Autodesk Fusion 360 part; units mm, degrees
(part 4 of 5)
  spline S117 degree 5 poles (-17.8005, -20.6587) (-17.8021, -20.6614) (-17.8082, -20.6716) (-17.8187, -20.6895) (-17.8335, -20.715) (-17.8525, -20.7483) (-17.8741, -20.7867) (-17.8954, -20.8254) (-17.9164, -20.8642) (-17.9371, -20.9032) (-17.9576, -20.9425) (-17.9778, -20.9819) (-17.9978, -21.0215) (-18.0175, -21.0613) (-18.037, -21.1012) (-18.0562, -21.1414) (-18.0753, -21.1816) (-18.0941, -21.2221) (-18.1127, -21.2627) (-18.1311, -21.3034) (-18.1492, -21.3443) (-18.1672, -21.3853) (-18.1849, -21.4265) (-18.2025, -21.4679) (-18.2198, -21.5093) (-18.237, -21.5509) (-18.2539, -21.5926) (-18.2706, -21.6345) (-18.2872, -21.6765) (-18.3036, -21.7186) (-18.3198, -21.7608) (-18.3357, -21.8032) (-18.3516, -21.8457) (-18.3672, -21.8882) (-18.3826, -21.931) (-18.3979, -21.9738) (-18.413, -22.0167) (-18.4279, -22.0598) (-18.4426, -22.103) (-18.4571, -22.1462) (-18.4715, -22.1896) (-18.4857, -22.2331) (-18.4998, -22.2767) (-18.5136, -22.3204) (-18.5273, -22.3642) (-18.5409, -22.4081) (-18.5542, -22.4521) (-18.5674, -22.4962) (-18.5805, -22.5404) (-18.5933, -22.5847) (-18.606, -22.6291) (-18.6186, -22.6736) (-18.6309, -22.7182) (-18.6432, -22.7628) (-18.6552, -22.8076) (-18.6671, -22.8525) (-18.6789, -22.8974) (-18.6904, -22.9424) (-18.7019, -22.9876) (-18.7131, -23.0328) (-18.7243, -23.0781) (-18.7352, -23.1235) (-18.7439, -23.1598) (-18.7503, -23.1871) (-18.7545, -23.2054) (-18.7566, -23.2145) knots 0.13777296 0.13777296 0.13777296 0.13777296 0.13777296 0.13777296 0.14285714 0.15714286 0.17142857 0.18571429 0.2 0.21428571 0.22857143 0.24285714 0.25714286 0.27142857 0.28571429 0.3 0.31428571 0.32857143 0.34285714 0.35714286 0.37142857 0.38571429 0.4 0.41428571 0.42857143 0.44285714 0.45714286 0.47142857 0.48571429 0.5 0.51428571 0.52857143 0.54285714 0.55714286 0.57142857 0.58571429 0.6 0.61428571 0.62857143 0.64285714 0.65714286 0.67142857 0.68571429 0.7 0.71428571 0.72857143 0.74285714 0.75714286 0.77142857 0.78571429 0.8 0.81428571 0.82857143 0.84285714 0.85714286 0.87142857 0.88571429 0.9 0.91428571 0.92857143 0.94285714 0.95714286 0.97142857 0.98571429 1 1 1 1 1 1
  arc A59 (-18.7566, -23.2145) -> (-17.9873, -23.8156) centre (0, 0) ccw
  spline S118 degree 5 poles (-17.9873, -23.8156) (-17.9789, -23.8113) (-17.9623, -23.8028) (-17.9373, -23.79) (-17.9041, -23.7728) (-17.8627, -23.7512) (-17.8215, -23.7294) (-17.7803, -23.7075) (-17.7393, -23.6855) (-17.6984, -23.6634) (-17.6577, -23.6411) (-17.617, -23.6187) (-17.5765, -23.5962) (-17.5361, -23.5735) (-17.4958, -23.5508) (-17.4557, -23.5278) (-17.4157, -23.5048) (-17.3758, -23.4816) (-17.3361, -23.4582) (-17.2965, -23.4347) (-17.257, -23.4111) (-17.2177, -23.3874) (-17.1785, -23.3635) (-17.1395, -23.3395) (-17.1006, -23.3153) (-17.0618, -23.291) (-17.0232, -23.2665) (-16.9847, -23.242) (-16.9464, -23.2172) (-16.9082, -23.1923) (-16.8702, -23.1673) (-16.8324, -23.1422) (-16.7947, -23.1168) (-16.7571, -23.0914) (-16.7197, -23.0658) (-16.6825, -23.04) (-16.6454, -23.0141) (-16.6085, -22.988) (-16.5718, -22.9618) (-16.5352, -22.9354) (-16.4988, -22.9089) (-16.4626, -22.8822) (-16.4266, -22.8553) (-16.3907, -22.8283) (-16.3551, -22.8011) (-16.3196, -22.7738) (-16.2843, -22.7463) (-16.2492, -22.7186) (-16.2143, -22.6907) (-16.1797, -22.6627) (-16.1452, -22.6345) (-16.1109, -22.6061) (-16.0769, -22.5775) (-16.043, -22.5487) (-16.0094, -22.5198) (-15.976, -22.4906) (-15.9429, -22.4613) (-15.9101, -22.4317) (-15.8775, -22.4019) (-15.8451, -22.3719) (-15.8131, -22.3417) (-15.7854, -22.3152) (-15.7642, -22.2946) (-15.7494, -22.2801) (-15.7409, -22.2718) (-15.7387, -22.2696) knots -1 -1 -1 -1 -1 -1 -0.98571429 -0.97142857 -0.95714286 -0.94285714 -0.92857143 -0.91428571 -0.9 -0.88571429 -0.87142857 -0.85714286 -0.84285714 -0.82857143 -0.81428571 -0.8 -0.78571429 -0.77142857 -0.75714286 -0.74285714 -0.72857143 -0.71428571 -0.7 -0.68571429 -0.67142857 -0.65714286 -0.64285714 -0.62857143 -0.61428571 -0.6 -0.58571429 -0.57142857 -0.55714286 -0.54285714 -0.52857143 -0.51428571 -0.5 -0.48571429 -0.47142857 -0.45714286 -0.44285714 -0.42857143 -0.41428571 -0.4 -0.38571429 -0.37142857 -0.35714286 -0.34285714 -0.32857143 -0.31428571 -0.3 -0.28571429 -0.27142857 -0.25714286 -0.24285714 -0.22857143 -0.21428571 -0.2 -0.18571429 -0.17142857 -0.15714286 -0.14285714 -0.13777296 -0.13777296 -0.13777296 -0.13777296 -0.13777296 -0.13777296
  spline S119 degree 3 poles (-15.4839, -22.2477) (-15.5053, -22.2329) (-15.5294, -22.2223) (-15.5802, -22.211) (-15.6065, -22.2104) (-15.6522, -22.2183) (-15.6716, -22.2247) (-15.7077, -22.2433) (-15.7242, -22.2553) (-15.7387, -22.2696) knots 0 0 0 0 0.007813 0.007813 0.015626 0.015626 0.021719 0.021719 0.027811 0.027811 0.027811 0.027811
  arc A60 (-15.4839, -22.2477) -> (-14.8274, -22.6906) centre (0, 0) ccw
  spline S120 degree 3 poles (-14.7522, -22.935) (-14.7421, -22.9109) (-14.7369, -22.8852) (-14.7366, -22.8331) (-14.7416, -22.8073) (-14.7589, -22.7643) (-14.7693, -22.7467) (-14.7951, -22.7154) (-14.8104, -22.7017) (-14.8274, -22.6906) knots 0 0 0 0 0.007813 0.007813 0.015626 0.015626 0.021719 0.021719 0.027811 0.027811 0.027811 0.027811
  spline S121 degree 5 poles (-14.7522, -22.935) (-14.7534, -22.9379) (-14.7579, -22.9489) (-14.7658, -22.968) (-14.7769, -22.9954) (-14.7912, -23.031) (-14.8072, -23.072) (-14.8229, -23.1132) (-14.8383, -23.1546) (-14.8534, -23.1962) (-14.8682, -23.2379) (-14.8827, -23.2797) (-14.897, -23.3217) (-14.911, -23.3639) (-14.9247, -23.4062) (-14.9382, -23.4486) (-14.9515, -23.4911) (-14.9645, -23.5338) (-14.9772, -23.5765) (-14.9898, -23.6194) (-15.0021, -23.6625) (-15.0141, -23.7056) (-15.026, -23.7489) (-15.0376, -23.7922) (-15.049, -23.8357) (-15.0602, -23.8793) (-15.0711, -23.9229) (-15.0819, -23.9667) (-15.0925, -24.0106) (-15.1028, -24.0546) (-15.1129, -24.0987) (-15.1229, -24.1428) (-15.1326, -24.1871) (-15.1422, -24.2314) (-15.1515, -24.2759) (-15.1607, -24.3204) (-15.1696, -24.3651) (-15.1784, -24.4098) (-15.187, -24.4546) (-15.1954, -24.4994) (-15.2036, -24.5444) (-15.2116, -24.5894) (-15.2194, -24.6346) (-15.2271, -24.6798) (-15.2345, -24.7251) (-15.2418, -24.7704) (-15.2489, -24.8158) (-15.2559, -24.8614) (-15.2626, -24.9069) (-15.2692, -24.9526) (-15.2756, -24.9983) (-15.2818, -25.0441) (-15.2879, -25.09) (-15.2938, -25.1359) (-15.2995, -25.1819) (-15.305, -25.228) (-15.3104, -25.2742) (-15.3156, -25.3204) (-15.3206, -25.3666) (-15.3255, -25.413) (-15.3302, -25.4594) (-15.3347, -25.5059) (-15.3382, -25.5431) (-15.3408, -25.571) (-15.3424, -25.5897) (-15.3433, -25.599) knots 0.13777296 0.13777296 0.13777296 0.13777296 0.13777296 0.13777296 0.14285714 0.15714286 0.17142857 0.18571429 0.2 0.21428571 0.22857143 0.24285714 0.25714286 0.27142857 0.28571429 0.3 0.31428571 0.32857143 0.34285714 0.35714286 0.37142857 0.38571429 0.4 0.41428571 0.42857143 0.44285714 0.45714286 0.47142857 0.48571429 0.5 0.51428571 0.52857143 0.54285714 0.55714286 0.57142857 0.58571429 0.6 0.61428571 0.62857143 0.64285714 0.65714286 0.67142857 0.68571429 0.7 0.71428571 0.72857143 0.74285714 0.75714286 0.77142857 0.78571429 0.8 0.81428571 0.82857143 0.84285714 0.85714286 0.87142857 0.88571429 0.9 0.91428571 0.92857143 0.94285714 0.95714286 0.97142857 0.98571429 1 1 1 1 1 1
  arc A61 (-15.3433, -25.599) -> (-14.4977, -26.0871) centre (0, 0) ccw
  spline S122 degree 5 poles (-14.4977, -26.0871) (-14.4901, -26.0818) (-14.4748, -26.071) (-14.4518, -26.0548) (-14.4214, -26.0332) (-14.3834, -26.006) (-14.3455, -25.9788) (-14.3079, -25.9514) (-14.2703, -25.9239) (-14.2329, -25.8963) (-14.1956, -25.8685) (-14.1585, -25.8407) (-14.1215, -25.8128) (-14.0846, -25.7847) (-14.0479, -25.7565) (-14.0114, -25.7282) (-13.975, -25.6998) (-13.9387, -25.6713) (-13.9026, -25.6426) (-13.8667, -25.6139) (-13.8309, -25.585) (-13.7953, -25.556) (-13.7598, -25.5269) (-13.7245, -25.4977) (-13.6893, -25.4683) (-13.6543, -25.4389) (-13.6195, -25.4093) (-13.5848, -25.3796) (-13.5503, -25.3498) (-13.5159, -25.3198) (-13.4818, -25.2897) (-13.4478, -25.2595) (-13.414, -25.2292) (-13.3803, -25.1988) (-13.3469, -25.1682) (-13.3136, -25.1375) (-13.2805, -25.1067) (-13.2476, -25.0758) (-13.2148, -25.0447) (-13.1823, -25.0135) (-13.15, -24.9821) (-13.1178, -24.9506) (-13.0859, -24.919) (-13.0541, -24.8873) (-13.0226, -24.8554) (-12.9913, -24.8234) (-12.9602, -24.7912) (-12.9293, -24.7589) (-12.8986, -24.7265) (-12.8682, -24.6939) (-12.8379, -24.6611) (-12.808, -24.6283) (-12.7782, -24.5952) (-12.7487, -24.562) (-12.7195, -24.5287) (-12.6905, -24.4952) (-12.6618, -24.4615) (-12.6333, -24.4276) (-12.6052, -24.3936) (-12.5774, -24.3594) (-12.5498, -24.325) (-12.5261, -24.2949) (-12.508, -24.2716) (-12.4953, -24.2552) (-12.4881, -24.2457) (-12.4862, -24.2432) knots -1 -1 -1 -1 -1 -1 -0.98571429 -0.97142857 -0.95714286 -0.94285714 -0.92857143 -0.91428571 -0.9 -0.88571429 -0.87142857 -0.85714286 -0.84285714 -0.82857143 -0.81428571 -0.8 -0.78571429 -0.77142857 -0.75714286 -0.74285714 -0.72857143 -0.71428571 -0.7 -0.68571429 -0.67142857 -0.65714286 -0.64285714 -0.62857143 -0.61428571 -0.6 -0.58571429 -0.57142857 -0.55714286 -0.54285714 -0.52857143 -0.51428571 -0.5 -0.48571429 -0.47142857 -0.45714286 -0.44285714 -0.42857143 -0.41428571 -0.4 -0.38571429 -0.37142857 -0.35714286 -0.34285714 -0.32857143 -0.31428571 -0.3 -0.28571429 -0.27142857 -0.25714286 -0.24285714 -0.22857143 -0.21428571 -0.2 -0.18571429 -0.17142857 -0.15714286 -0.14285714 -0.13777296 -0.13777296 -0.13777296 -0.13777296 -0.13777296 -0.13777296
  spline S123 degree 3 poles (-12.237, -24.1862) (-12.2602, -24.1744) (-12.2855, -24.1673) (-12.3374, -24.1632) (-12.3636, -24.1662) (-12.4077, -24.1804) (-12.426, -24.1895) (-12.4592, -24.2129) (-12.4739, -24.2271) (-12.4862, -24.2432) knots 0 0 0 0 0.007813 0.007813 0.015626 0.015626 0.021719 0.021719 0.027811 0.027811 0.027811 0.027811
  arc A62 (-12.237, -24.1862) -> (-11.5251, -24.5334) centre (0, 0) ccw
  spline S124 degree 3 poles (-11.4167, -24.7649) (-11.4101, -24.7397) (-11.4085, -24.7134) (-11.4154, -24.6618) (-11.4239, -24.6369) (-11.4471, -24.5968) (-11.4599, -24.5809) (-11.4898, -24.5534) (-11.5067, -24.542) (-11.5251, -24.5334) knots 0 0 0 0 0.007813 0.007813 0.015626 0.015626 0.021719 0.021719 0.027811 0.027811 0.027811 0.027811
  spline S125 degree 5 poles (-11.4167, -24.7649) (-11.4174, -24.7679) (-11.4204, -24.7794) (-11.4256, -24.7995) (-11.4328, -24.8281) (-11.4419, -24.8654) (-11.4521, -24.9082) (-11.4619, -24.9512) (-11.4714, -24.9944) (-11.4806, -25.0376) (-11.4894, -25.081) (-11.498, -25.1244) (-11.5063, -25.168) (-11.5142, -25.2117) (-11.522, -25.2555) (-11.5294, -25.2994) (-11.5366, -25.3433) (-11.5436, -25.3874) (-11.5502, -25.4315) (-11.5567, -25.4758) (-11.5629, -25.5201) (-11.5688, -25.5645) (-11.5745, -25.6089) (-11.58, -25.6535) (-11.5852, -25.6981) (-11.5902, -25.7428) (-11.595, -25.7876) (-11.5996, -25.8325) (-11.6039, -25.8774) (-11.6081, -25.9224) (-11.612, -25.9674) (-11.6157, -26.0126) (-11.6192, -26.0578) (-11.6224, -26.103) (-11.6255, -26.1483) (-11.6284, -26.1937) (-11.631, -26.2391) (-11.6335, -26.2846) (-11.6358, -26.3302) (-11.6378, -26.3758) (-11.6397, -26.4215) (-11.6414, -26.4672) (-11.6428, -26.513) (-11.6441, -26.5588) (-11.6452, -26.6047) (-11.6461, -26.6506) (-11.6468, -26.6966) (-11.6474, -26.7426) (-11.6477, -26.7887) (-11.6479, -26.8348) (-11.6478, -26.881) (-11.6476, -26.9272) (-11.6472, -26.9735) (-11.6467, -27.0198) (-11.6459, -27.0662) (-11.645, -27.1125) (-11.6439, -27.159) (-11.6426, -27.2055) (-11.6412, -27.252) (-11.6395, -27.2986) (-11.6377, -27.3452) (-11.6358, -27.3918) (-11.634, -27.4292) (-11.6327, -27.4572) (-11.6317, -27.4759) (-11.6312, -27.4852) knots 0.13777296 0.13777296 0.13777296 0.13777296 0.13777296 0.13777296 0.14285714 0.15714286 0.17142857 0.18571429 0.2 0.21428571 0.22857143 0.24285714 0.25714286 0.27142857 0.28571429 0.3 0.31428571 0.32857143 0.34285714 0.35714286 0.37142857 0.38571429 0.4 0.41428571 0.42857143 0.44285714 0.45714286 0.47142857 0.48571429 0.5 0.51428571 0.52857143 0.54285714 0.55714286 0.57142857 0.58571429 0.6 0.61428571 0.62857143 0.64285714 0.65714286 0.67142857 0.68571429 0.7 0.71428571 0.72857143 0.74285714 0.75714286 0.77142857 0.78571429 0.8 0.81428571 0.82857143 0.84285714 0.85714286 0.87142857 0.88571429 0.9 0.91428571 0.92857143 0.94285714 0.95714286 0.97142857 0.98571429 1 1 1 1 1 1
  arc A63 (-11.6312, -27.4852) -> (-10.726, -27.851) centre (0, 0) ccw
  spline S126 degree 5 poles (-10.726, -27.851) (-10.7192, -27.8446) (-10.7055, -27.8318) (-10.6851, -27.8126) (-10.6579, -27.7869) (-10.6241, -27.7547) (-10.5904, -27.7224) (-10.5569, -27.6901) (-10.5235, -27.6576) (-10.4903, -27.6251) (-10.4572, -27.5924) (-10.4243, -27.5597) (-10.3916, -27.5269) (-10.359, -27.494) (-10.3266, -27.4609) (-10.2944, -27.4278) (-10.2623, -27.3946) (-10.2303, -27.3613) (-10.1986, -27.328) (-10.167, -27.2945) (-10.1355, -27.2609) (-10.1043, -27.2272) (-10.0732, -27.1935) (-10.0423, -27.1596) (-10.0116, -27.1257) (-9.981, -27.0916) (-9.9506, -27.0575) (-9.9204, -27.0232) (-9.8904, -26.9889) (-9.8606, -26.9545) (-9.8309, -26.9199) (-9.8015, -26.8853) (-9.7722, -26.8506) (-9.7431, -26.8157) (-9.7142, -26.7808) (-9.6855, -26.7458) (-9.6571, -26.7107) (-9.6288, -26.6754) (-9.6007, -26.6401) (-9.5728, -26.6047) (-9.5452, -26.5691) (-9.5177, -26.5335) (-9.4905, -26.4977) (-9.4635, -26.4619) (-9.4367, -26.4259) (-9.4101, -26.3898) (-9.3838, -26.3537) (-9.3577, -26.3174) (-9.3318, -26.281) (-9.3062, -26.2445) (-9.2808, -26.2078) (-9.2557, -26.1711) (-9.2309, -26.1342) (-9.2063, -26.0973) (-9.1819, -26.0602) (-9.1579, -26.023) (-9.1342, -25.9856) (-9.1107, -25.9481) (-9.0876, -25.9105) (-9.0648, -25.8728) (-9.0423, -25.8349) (-9.023, -25.8017) (-9.0083, -25.7762) (-8.9981, -25.7581) (-8.9922, -25.7478) (-8.9907, -25.745) knots -1 -1 -1 -1 -1 -1 -0.98571429 -0.97142857 -0.95714286 -0.94285714 -0.92857143 -0.91428571 -0.9 -0.88571429 -0.87142857 -0.85714286 -0.84285714 -0.82857143 -0.81428571 -0.8 -0.78571429 -0.77142857 -0.75714286 -0.74285714 -0.72857143 -0.71428571 -0.7 -0.68571429 -0.67142857 -0.65714286 -0.64285714 -0.62857143 -0.61428571 -0.6 -0.58571429 -0.57142857 -0.55714286 -0.54285714 -0.52857143 -0.51428571 -0.5 -0.48571429 -0.47142857 -0.45714286 -0.44285714 -0.42857143 -0.41428571 -0.4 -0.38571429 -0.37142857 -0.35714286 -0.34285714 -0.32857143 -0.31428571 -0.3 -0.28571429 -0.27142857 -0.25714286 -0.24285714 -0.22857143 -0.21428571 -0.2 -0.18571429 -0.17142857 -0.15714286 -0.14285714 -0.13777296 -0.13777296 -0.13777296 -0.13777296 -0.13777296 -0.13777296
  spline S127 degree 3 poles (-8.7518, -25.6538) (-8.7765, -25.6454) (-8.8025, -25.6419) (-8.8545, -25.6451) (-8.8799, -25.6517) (-8.9217, -25.6719) (-8.9385, -25.6835) (-8.9681, -25.7113) (-8.9807, -25.7273) (-8.9907, -25.745) knots 0 0 0 0 0.007813 0.007813 0.015626 0.015626 0.021719 0.021719 0.027811 0.027811 0.027811 0.027811
  arc A64 (-8.7518, -25.6538) -> (-7.9986, -25.8986) centre (0, 0) ccw
  spline S128 degree 3 poles (-7.8589, -26.1128) (-7.8559, -26.0869) (-7.858, -26.0607) (-7.8721, -26.0105) (-7.884, -25.9871) (-7.9125, -25.9506) (-7.9274, -25.9365) (-7.9608, -25.9135) (-7.9792, -25.9046) (-7.9986, -25.8986) knots 0 0 0 0 0.007813 0.007813 0.015626 0.015626 0.021719 0.021719 0.027811 0.027811 0.027811 0.027811
  spline S129 degree 5 poles (-7.8589, -26.1128) (-7.8593, -26.1159) (-7.8607, -26.1277) (-7.863, -26.1483) (-7.8661, -26.1776) (-7.87, -26.2158) (-7.874, -26.2597) (-7.8778, -26.3036) (-7.8812, -26.3476) (-7.8843, -26.3917) (-7.887, -26.4359) (-7.8894, -26.4801) (-7.8916, -26.5245) (-7.8934, -26.5688) (-7.8949, -26.6132) (-7.8962, -26.6577) (-7.8972, -26.7023) (-7.898, -26.7469) (-7.8985, -26.7915) (-7.8987, -26.8362) (-7.8986, -26.881) (-7.8983, -26.9257) (-7.8978, -26.9706) (-7.897, -27.0155) (-7.896, -27.0604) (-7.8947, -27.1054) (-7.8933, -27.1504) (-7.8915, -27.1954) (-7.8896, -27.2405) (-7.8874, -27.2856) (-7.885, -27.3308) (-7.8824, -27.376) (-7.8796, -27.4212) (-7.8765, -27.4665) (-7.8732, -27.5118) (-7.8698, -27.5571) (-7.8661, -27.6025) (-7.8622, -27.6479) (-7.8581, -27.6933) (-7.8538, -27.7388) (-7.8493, -27.7843) (-7.8445, -27.8298) (-7.8396, -27.8753) (-7.8345, -27.9209) (-7.8292, -27.9665) (-7.8237, -28.0121) (-7.818, -28.0577) (-7.8122, -28.1034) (-7.8061, -28.149) (-7.7998, -28.1947) (-7.7934, -28.2405) (-7.7867, -28.2862) (-7.7799, -28.332) (-7.7729, -28.3777) (-7.7657, -28.4235) (-7.7583, -28.4694) (-7.7508, -28.5152) (-7.743, -28.5611) (-7.7351, -28.6069) (-7.727, -28.6528) (-7.7188, -28.6987) (-7.7103, -28.7446) (-7.7034, -28.7814) (-7.6982, -28.8089) (-7.6946, -28.8273) (-7.6928, -28.8365) knots 0.13777296 0.13777296 0.13777296 0.13777296 0.13777296 0.13777296 0.14285714 0.15714286 0.17142857 0.18571429 0.2 0.21428571 0.22857143 0.24285714 0.25714286 0.27142857 0.28571429 0.3 0.31428571 0.32857143 0.34285714 0.35714286 0.37142857 0.38571429 0.4 0.41428571 0.42857143 0.44285714 0.45714286 0.47142857 0.48571429 0.5 0.51428571 0.52857143 0.54285714 0.55714286 0.57142857 0.58571429 0.6 0.61428571 0.62857143 0.64285714 0.65714286 0.67142857 0.68571429 0.7 0.71428571 0.72857143 0.74285714 0.75714286 0.77142857 0.78571429 0.8 0.81428571 0.82857143 0.84285714 0.85714286 0.87142857 0.88571429 0.9 0.91428571 0.92857143 0.94285714 0.95714286 0.97142857 0.98571429 1 1 1 1 1 1
  arc A65 (-7.6928, -28.8365) -> (-6.7455, -29.0727) centre (0, 0) ccw
  spline S130 degree 5 poles (-6.7455, -29.0727) (-6.7397, -29.0654) (-6.7279, -29.0508) (-6.7103, -29.029) (-6.687, -28.9998) (-6.658, -28.9632) (-6.6291, -28.9266) (-6.6004, -28.8898) (-6.5719, -28.8531) (-6.5435, -28.8162) (-6.5154, -28.7793) (-6.4873, -28.7423) (-6.4595, -28.7052) (-6.4318, -28.6681) (-6.4043, -28.6309) (-6.377, -28.5936) (-6.3498, -28.5563) (-6.3228, -28.5189) (-6.296, -28.4814) (-6.2694, -28.4438) (-6.2429, -28.4062) (-6.2167, -28.3685) (-6.1906, -28.3308) (-6.1647, -28.2929) (-6.139, -28.255) (-6.1134, -28.2171) (-6.0881, -28.179) (-6.063, -28.1409) (-6.038, -28.1027) (-6.0133, -28.0645) (-5.9887, -28.0261) (-5.9644, -27.9877) (-5.9402, -27.9493) (-5.9163, -27.9107) (-5.8925, -27.8721) (-5.869, -27.8335) (-5.8457, -27.7947) (-5.8226, -27.7559) (-5.7997, -27.717) (-5.777, -27.678) (-5.7546, -27.639) (-5.7323, -27.5999) (-5.7103, -27.5607) (-5.6886, -27.5214) (-5.667, -27.4821) (-5.6458, -27.4427) (-5.6247, -27.4032) (-5.6039, -27.3636) (-5.5834, -27.324) (-5.5631, -27.2842) (-5.5431, -27.2444) (-5.5233, -27.2046) (-5.5039, -27.1646) (-5.4846, -27.1246) (-5.4657, -27.0844) (-5.4471, -27.0442) (-5.4288, -27.004) (-5.4108, -26.9636) (-5.3931, -26.9231) (-5.3758, -26.8825) (-5.3588, -26.8419) (-5.3443, -26.8064) (-5.3333, -26.779) (-5.3257, -26.7598) (-5.3213, -26.7487) (-5.3202, -26.7458) knots -1 -1 -1 -1 -1 -1 -0.98571429 -0.97142857 -0.95714286 -0.94285714 -0.92857143 -0.91428571 -0.9 -0.88571429 -0.87142857 -0.85714286 -0.84285714 -0.82857143 -0.81428571 -0.8 -0.78571429 -0.77142857 -0.75714286 -0.74285714 -0.72857143 -0.71428571 -0.7 -0.68571429 -0.67142857 -0.65714286 -0.64285714 -0.62857143 -0.61428571 -0.6 -0.58571429 -0.57142857 -0.55714286 -0.54285714 -0.52857143 -0.51428571 -0.5 -0.48571429 -0.47142857 -0.45714286 -0.44285714 -0.42857143 -0.41428571 -0.4 -0.38571429 -0.37142857 -0.35714286 -0.34285714 -0.32857143 -0.31428571 -0.3 -0.28571429 -0.27142857 -0.25714286 -0.24285714 -0.22857143 -0.21428571 -0.2 -0.18571429 -0.17142857 -0.15714286 -0.14285714 -0.13777296 -0.13777296 -0.13777296 -0.13777296 -0.13777296 -0.13777296
  spline S131 degree 3 poles (-5.0963, -26.6222) (-5.1219, -26.6173) (-5.1482, -26.6175) (-5.1992, -26.6278) (-5.2235, -26.6379) (-5.262, -26.6637) (-5.2771, -26.6775) (-5.3025, -26.7092) (-5.3128, -26.7268) (-5.3202, -26.7458) knots 0 0 0 0 0.007813 0.007813 0.015626 0.015626 0.021719 0.021719 0.027811 0.027811 0.027811 0.027811
  arc A66 (-5.0963, -26.6222) -> (-4.3164, -26.7597) centre (0, 0) ccw
  spline S132 degree 3 poles (-4.1483, -26.9524) (-4.1489, -26.9264) (-4.1546, -26.9007) (-4.1755, -26.853) (-4.1905, -26.8314) (-4.2239, -26.7992) (-4.2405, -26.7874) (-4.2769, -26.7692) (-4.2963, -26.763) (-4.3164, -26.7597) knots 0 0 0 0 0.007813 0.007813 0.015626 0.015626 0.021719 0.021719 0.027811 0.027811 0.027811 0.027811
  spline S133 degree 5 poles (-4.1483, -26.9524) (-4.1482, -26.9555) (-4.1479, -26.9674) (-4.1473, -26.9881) (-4.1464, -27.0176) (-4.1449, -27.0559) (-4.1428, -27.1) (-4.1404, -27.144) (-4.1376, -27.1881) (-4.1345, -27.2322) (-4.1311, -27.2763) (-4.1273, -27.3204) (-4.1233, -27.3646) (-4.1189, -27.4088) (-4.1143, -27.453) (-4.1093, -27.4972) (-4.1041, -27.5415) (-4.0987, -27.5858) (-4.0929, -27.63) (-4.0869, -27.6743) (-4.0807, -27.7186) (-4.0741, -27.7629) (-4.0674, -27.8073) (-4.0603, -27.8516) (-4.0531, -27.896) (-4.0456, -27.9403) (-4.0378, -27.9847) (-4.0299, -28.0291) (-4.0217, -28.0734) (-4.0132, -28.1178) (-4.0046, -28.1622) (-3.9957, -28.2066) (-3.9866, -28.251) (-3.9772, -28.2954) (-3.9677, -28.3398) (-3.958, -28.3842) (-3.948, -28.4286) (-3.9378, -28.473) (-3.9274, -28.5175) (-3.9168, -28.5619) (-3.906, -28.6063) (-3.895, -28.6507) (-3.8838, -28.6951) (-3.8725, -28.7395) (-3.8609, -28.7839) (-3.8491, -28.8283) (-3.8371, -28.8727) (-3.8249, -28.9171) (-3.8125, -28.9615) (-3.8, -29.0059) (-3.7872, -29.0502) (-3.7743, -29.0946) (-3.7611, -29.139) (-3.7478, -29.1834) (-3.7343, -29.2277) (-3.7207, -29.2721) (-3.7068, -29.3164) (-3.6928, -29.3607) (-3.6785, -29.405) (-3.6641, -29.4494) (-3.6496, -29.4937) (-3.6348, -29.538) (-3.6229, -29.5734) (-3.6138, -29.5999) (-3.6078, -29.6177) (-3.6047, -29.6265) knots 0.13777296 0.13777296 0.13777296 0.13777296 0.13777296 0.13777296 0.14285714 0.15714286 0.17142857 0.18571429 0.2 0.21428571 0.22857143 0.24285714 0.25714286 0.27142857 0.28571429 0.3 0.31428571 0.32857143 0.34285714 0.35714286 0.37142857 0.38571429 0.4 0.41428571 0.42857143 0.44285714 0.45714286 0.47142857 0.48571429 0.5 0.51428571 0.52857143 0.54285714 0.55714286 0.57142857 0.58571429 0.6 0.61428571 0.62857143 0.64285714 0.65714286 0.67142857 0.68571429 0.7 0.71428571 0.72857143 0.74285714 0.75714286 0.77142857 0.78571429 0.8 0.81428571 0.82857143 0.84285714 0.85714286 0.87142857 0.88571429 0.9 0.91428571 0.92857143 0.94285714 0.95714286 0.97142857 0.98571429 1 1 1 1 1 1
  arc A67 (-3.6047, -29.6265) -> (-2.6338, -29.7286) centre (0, 0) ccw
  spline S134 degree 5 poles (-2.6338, -29.7286) (-2.6289, -29.7205) (-2.6193, -29.7045) (-2.605, -29.6804) (-2.5859, -29.6482) (-2.5623, -29.6079) (-2.5388, -29.5676) (-2.5155, -29.5273) (-2.4924, -29.4869) (-2.4694, -29.4464) (-2.4466, -29.406) (-2.424, -29.3654) (-2.4016, -29.3248) (-2.3794, -29.2842) (-2.3573, -29.2436) (-2.3354, -29.2028) (-2.3137, -29.1621) (-2.2922, -29.1213) (-2.2709, -29.0804) (-2.2497, -29.0395) (-2.2288, -28.9986) (-2.208, -28.9576) (-2.1874, -28.9166) (-2.1671, -28.8755) (-2.1469, -28.8344) (-2.1269, -28.7933) (-2.1071, -28.7521) (-2.0875, -28.7108) (-2.0681, -28.6696) (-2.0489, -28.6282) (-2.03, -28.5869) (-2.0112, -28.5455) (-1.9926, -28.504) (-1.9743, -28.4625) (-1.9561, -28.421) (-1.9382, -28.3794) (-1.9205, -28.3378) (-1.903, -28.2961) (-1.8858, -28.2544) (-1.8687, -28.2127) (-1.852, -28.1709) (-1.8354, -28.129) (-1.8191, -28.0872) (-1.803, -28.0453) (-1.7871, -28.0033) (-1.7715, -27.9613) (-1.7562, -27.9193) (-1.7411, -27.8772) (-1.7263, -27.8351) (-1.7117, -27.7929) (-1.6975, -27.7507) (-1.6834, -27.7085) (-1.6697, -27.6662) (-1.6563, -27.6239) (-1.6431, -27.5815) (-1.6302, -27.5391) (-1.6177, -27.4967) (-1.6055, -27.4542) (-1.5937, -27.4117) (-1.5821, -27.3691) (-1.571, -27.3265) (-1.5615, -27.2893) (-1.5545, -27.2607) (-1.5496, -27.2405) (-1.5468, -27.2289) (-1.5461, -27.2259) knots -1 -1 -1 -1 -1 -1 -0.98571429 -0.97142857 -0.95714286 -0.94285714 -0.92857143 -0.91428571 -0.9 -0.88571429 -0.87142857 -0.85714286 -0.84285714 -0.82857143 -0.81428571 -0.8 -0.78571429 -0.77142857 -0.75714286 -0.74285714 -0.72857143 -0.71428571 -0.7 -0.68571429 -0.67142857 -0.65714286 -0.64285714 -0.62857143 -0.61428571 -0.6 -0.58571429 -0.57142857 -0.55714286 -0.54285714 -0.52857143 -0.51428571 -0.5 -0.48571429 -0.47142857 -0.45714286 -0.44285714 -0.42857143 -0.41428571 -0.4 -0.38571429 -0.37142857 -0.35714286 -0.34285714 -0.32857143 -0.31428571 -0.3 -0.28571429 -0.27142857 -0.25714286 -0.24285714 -0.22857143 -0.21428571 -0.2 -0.18571429 -0.17142857 -0.15714286 -0.14285714 -0.13777296 -0.13777296 -0.13777296 -0.13777296 -0.13777296 -0.13777296
  spline S135 degree 3 poles (-1.3416, -27.0724) (-1.3676, -27.0711) (-1.3937, -27.0749) (-1.4428, -27.0923) (-1.4654, -27.1057) (-1.4999, -27.1365) (-1.5129, -27.1523) (-1.5337, -27.1872) (-1.5414, -27.2061) (-1.5461, -27.2259) knots 0 0 0 0 0.007813 0.007813 0.015626 0.015626 0.021719 0.021719 0.027811 0.027811 0.027811 0.027811
  arc A68 (-1.3416, -27.0724) -> (-0.5501, -27.1) centre (0, 0) ccw
  spline S136 degree 3 poles (-0.3568, -27.2674) (-0.3611, -27.2417) (-0.3703, -27.2171) (-0.3977, -27.1728) (-0.4155, -27.1535) (-0.453, -27.1263) (-0.4712, -27.1169) (-0.5097, -27.1039) (-0.5298, -27.1004) (-0.5501, -27.1) knots 0 0 0 0 0.007813 0.007813 0.015626 0.015626 0.021719 0.021719 0.027811 0.027811 0.027811 0.027811
  spline S137 degree 5 poles (-0.3568, -27.2674) (-0.3563, -27.2705) (-0.3544, -27.2823) (-0.3509, -27.3027) (-0.3459, -27.3318) (-0.3391, -27.3695) (-0.3309, -27.4128) (-0.3224, -27.4561) (-0.3135, -27.4993) (-0.3043, -27.5426) (-0.2948, -27.5858) (-0.2849, -27.629) (-0.2747, -27.6721) (-0.2643, -27.7153) (-0.2535, -27.7584) (-0.2425, -27.8016) (-0.2312, -27.8446) (-0.2196, -27.8877) (-0.2077, -27.9308) (-0.1956, -27.9738) (-0.1833, -28.0168) (-0.1706, -28.0598) (-0.1578, -28.1027) (-0.1446, -28.1457) (-0.1313, -28.1886) (-0.1177, -28.2314) (-0.1038, -28.2743) (-0.0897, -28.3171) (-0.0754, -28.3599) (-0.0609, -28.4027) (-0.0462, -28.4455) (-0.0312, -28.4882) (-0.016, -28.5309) (-0.0006, -28.5736) (0.015, -28.6162) (0.0309, -28.6588) (0.0469, -28.7014) (0.0632, -28.744) (0.0797, -28.7865) (0.0963, -28.829) (0.1132, -28.8715) (0.1303, -28.9139) (0.1475, -28.9564) (0.165, -28.9987) (0.1827, -29.0411) (0.2005, -29.0834) (0.2186, -29.1257) (0.2368, -29.168) (0.2552, -29.2102) (0.2739, -29.2524) (0.2927, -29.2946) (0.3116, -29.3368) (0.3308, -29.3789) (0.3502, -29.4209) (0.3697, -29.463) (0.3894, -29.505) (0.4093, -29.547) (0.4294, -29.5889) (0.4497, -29.6308) (0.4701, -29.6727) (0.4907, -29.7145) (0.5115, -29.7564) (0.5282, -29.7898) (0.5409, -29.8148) (0.5493, -29.8315) (0.5536, -29.8399) knots 0.13777296 0.13777296 0.13777296 0.13777296 0.13777296 0.13777296 0.14285714 0.15714286 0.17142857 0.18571429 0.2 0.21428571 0.22857143 0.24285714 0.25714286 0.27142857 0.28571429 0.3 0.31428571 0.32857143 0.34285714 0.35714286 0.37142857 0.38571429 0.4 0.41428571 0.42857143 0.44285714 0.45714286 0.47142857 0.48571429 0.5 0.51428571 0.52857143 0.54285714 0.55714286 0.57142857 0.58571429 0.6 0.61428571 0.62857143 0.64285714 0.65714286 0.67142857 0.68571429 0.7 0.71428571 0.72857143 0.74285714 0.75714286 0.77142857 0.78571429 0.8 0.81428571 0.82857143 0.84285714 0.85714286 0.87142857 0.88571429 0.9 0.91428571 0.92857143 0.94285714 0.95714286 0.97142857 0.98571429 1 1 1 1 1 1
  arc A69 (0.5536, -29.8399) -> (1.5293, -29.8058) centre (0, 0) ccw
  spline S138 degree 5 poles (1.5293, -29.8058) (1.5329, -29.7972) (1.5402, -29.7799) (1.5511, -29.7541) (1.5655, -29.7196) (1.5833, -29.6764) (1.6009, -29.6332) (1.6184, -29.59) (1.6357, -29.5468) (1.6528, -29.5036) (1.6697, -29.4603) (1.6864, -29.417) (1.703, -29.3737) (1.7194, -29.3304) (1.7355, -29.287) (1.7515, -29.2437) (1.7674, -29.2003) (1.783, -29.1569) (1.7984, -29.1135) (1.8137, -29.07) (1.8287, -29.0266) (1.8436, -28.9831) (1.8583, -28.9396) (1.8727, -28.8961) (1.887, -28.8526) (1.9011, -28.8091) (1.9149, -28.7655) (1.9286, -28.7219) (1.942, -28.6784) (1.9553, -28.6348) (1.9683, -28.5912) (1.9812, -28.5476) (1.9938, -28.5039) (2.0062, -28.4603) (2.0183, -28.4166) (2.0303, -28.373) (2.042, -28.3293) (2.0536, -28.2856) (2.0648, -28.2419) (2.0759, -28.1982) (2.0867, -28.1545) (2.0973, -28.1107) (2.1076, -28.067) (2.1177, -28.0233) (2.1276, -27.9795) (2.1372, -27.9358) (2.1465, -27.892) (2.1556, -27.8482) (2.1644, -27.8045) (2.1729, -27.7607) (2.1812, -27.7169) (2.1892, -27.6731) (2.1969, -27.6294) (2.2044, -27.5856) (2.2115, -27.5418) (2.2183, -27.498) (2.2248, -27.4542) (2.231, -27.4105) (2.2368, -27.3667) (2.2423, -27.3229) (2.2474, -27.2792) (2.2516, -27.2411) (2.2546, -27.2117) (2.2566, -27.1911) (2.2578, -27.1792) (2.2581, -27.1761) knots -1 -1 -1 -1 -1 -1 -0.98571429 -0.97142857 -0.95714286 -0.94285714 -0.92857143 -0.91428571 -0.9 -0.88571429 -0.87142857 -0.85714286 -0.84285714 -0.82857143 -0.81428571 -0.8 -0.78571429 -0.77142857 -0.75714286 -0.74285714 -0.72857143 -0.71428571 -0.7 -0.68571429 -0.67142857 -0.65714286 -0.64285714 -0.62857143 -0.61428571 -0.6 -0.58571429 -0.57142857 -0.55714286 -0.54285714 -0.52857143 -0.51428571 -0.5 -0.48571429 -0.47142857 -0.45714286 -0.44285714 -0.42857143 -0.41428571 -0.4 -0.38571429 -0.37142857 -0.35714286 -0.34285714 -0.32857143 -0.31428571 -0.3 -0.28571429 -0.27142857 -0.25714286 -0.24285714 -0.22857143 -0.21428571 -0.2 -0.18571429 -0.17142857 -0.15714286 -0.14285714 -0.13777296 -0.13777296 -0.13777296 -0.13777296 -0.13777296 -0.13777296
  spline S139 degree 3 poles (2.4392, -26.9956) (2.4132, -26.998) (2.388, -27.0054) (2.3418, -27.0294) (2.3213, -27.0458) (2.2913, -27.0812) (2.2807, -27.0986) (2.2649, -27.1361) (2.26, -27.1559) (2.2581, -27.1761) knots 0 0 0 0 0.007813 0.007813 0.015626 0.015626 0.021719 0.021719 0.027811 0.027811 0.027811 0.027811
  arc A70 (2.4392, -26.9956) -> (3.2268, -26.9129) centre (0, 0) ccw
  spline S140 degree 3 poles (3.4415, -27.0517) (3.4337, -27.0269) (3.4212, -27.0038) (3.3879, -26.9637) (3.3675, -26.9471) (3.3266, -26.9253) (3.3073, -26.9186) (3.2674, -26.9111) (3.247, -26.9104) (3.2268, -26.9129) knots 0 0 0 0 0.007813 0.007813 0.015626 0.015626 0.021719 0.021719 0.027811 0.027811 0.027811 0.027811
  spline S141 degree 5 poles (3.4415, -27.0517) (3.4425, -27.0547) (3.446, -27.0661) (3.4523, -27.0858) (3.4613, -27.1139) (3.4733, -27.1503) (3.4875, -27.1921) (3.5019, -27.2337) (3.5167, -27.2753) (3.5318, -27.3169) (3.5473, -27.3583) (3.5631, -27.3997) (3.5792, -27.4411) (3.5955, -27.4824) (3.6122, -27.5236) (3.6291, -27.5647) (3.6463, -27.6058) (3.6638, -27.6469) (3.6815, -27.6879) (3.6995, -27.7288) (3.7177, -27.7696) (3.7362, -27.8104) (3.7549, -27.8512) (3.7739, -27.8919) (3.7931, -27.9325) (3.8125, -27.9731) (3.8322, -28.0136) (3.8521, -28.054) (3.8722, -28.0944) (3.8926, -28.1348) (3.9131, -28.1751) (3.9339, -28.2153) (3.9549, -28.2555) (3.9761, -28.2956) (3.9975, -28.3356) (4.0191, -28.3756) (4.0409, -28.4156) (4.063, -28.4555) (4.0852, -28.4953) (4.1076, -28.5351) (4.1302, -28.5748) (4.153, -28.6144) (4.176, -28.654) (4.1992, -28.6936) (4.2226, -28.7331) (4.2462, -28.7725) (4.27, -28.8119) (4.2939, -28.8512) (4.318, -28.8904) (4.3423, -28.9296) (4.3668, -28.9688) (4.3915, -29.0079) (4.4163, -29.0469) (4.4414, -29.0859) (4.4666, -29.1248) (4.4919, -29.1637) (4.5175, -29.2025) (4.5432, -29.2412) (4.5691, -29.2799) (4.5951, -29.3185) (4.6214, -29.3571) (4.6478, -29.3956) (4.669, -29.4264) (4.685, -29.4494) (4.6957, -29.4647) (4.7011, -29.4724) knots 0.13777296 0.13777296 0.13777296 0.13777296 0.13777296 0.13777296 0.14285714 0.15714286 0.17142857 0.18571429 0.2 0.21428571 0.22857143 0.24285714 0.25714286 0.27142857 0.28571429 0.3 0.31428571 0.32857143 0.34285714 0.35714286 0.37142857 0.38571429 0.4 0.41428571 0.42857143 0.44285714 0.45714286 0.47142857 0.48571429 0.5 0.51428571 0.52857143 0.54285714 0.55714286 0.57142857 0.58571429 0.6 0.61428571 0.62857143 0.64285714 0.65714286 0.67142857 0.68571429 0.7 0.71428571 0.72857143 0.74285714 0.75714286 0.77142857 0.78571429 0.8 0.81428571 0.82857143 0.84285714 0.85714286 0.87142857 0.88571429 0.9 0.91428571 0.92857143 0.94285714 0.95714286 0.97142857 0.98571429 1 1 1 1 1 1
  arc A71 (4.7011, -29.4724) -> (5.6626, -29.3029) centre (0, 0) ccw
  spline S142 degree 5 poles (5.6626, -29.3029) (5.665, -29.2938) (5.6698, -29.2758) (5.677, -29.2486) (5.6864, -29.2124) (5.698, -29.1672) (5.7095, -29.122) (5.7208, -29.0768) (5.7319, -29.0316) (5.7428, -28.9864) (5.7535, -28.9412) (5.7641, -28.896) (5.7744, -28.8508) (5.7846, -28.8056) (5.7946, -28.7605) (5.8044, -28.7153) (5.8141, -28.6701) (5.8235, -28.625) (5.8327, -28.5798) (5.8418, -28.5347) (5.8506, -28.4896) (5.8593, -28.4445) (5.8678, -28.3994) (5.8761, -28.3543) (5.8841, -28.3092) (5.892, -28.2641) (5.8997, -28.2191) (5.9071, -28.174) (5.9144, -28.129) (5.9214, -28.084) (5.9283, -28.039) (5.9349, -27.994) (5.9413, -27.949) (5.9475, -27.9041) (5.9535, -27.8592) (5.9593, -27.8143) (5.9648, -27.7694) (5.9702, -27.7245) (5.9752, -27.6797) (5.9801, -27.6348) (5.9847, -27.5901) (5.9891, -27.5453) (5.9933, -27.5005) (5.9972, -27.4558) (6.0009, -27.4111) (6.0043, -27.3665) (6.0074, -27.3218) (6.0103, -27.2772) (6.013, -27.2326) (6.0153, -27.1881) (6.0174, -27.1436) (6.0193, -27.0991) (6.0208, -27.0547) (6.0221, -27.0103) (6.0231, -26.966) (6.0237, -26.9217) (6.0241, -26.8774) (6.0241, -26.8332) (6.0238, -26.7891) (6.0231, -26.745) (6.0221, -26.7009) (6.0209, -26.6626) (6.0198, -26.6331) (6.0189, -26.6124) (6.0184, -26.6005) (6.0183, -26.5974) knots -1 -1 -1 -1 -1 -1 -0.98571429 -0.97142857 -0.95714286 -0.94285714 -0.92857143 -0.91428571 -0.9 -0.88571429 -0.87142857 -0.85714286 -0.84285714 -0.82857143 -0.81428571 -0.8 -0.78571429 -0.77142857 -0.75714286 -0.74285714 -0.72857143 -0.71428571 -0.7 -0.68571429 -0.67142857 -0.65714286 -0.64285714 -0.62857143 -0.61428571 -0.6 -0.58571429 -0.57142857 -0.55714286 -0.54285714 -0.52857143 -0.51428571 -0.5 -0.48571429 -0.47142857 -0.45714286 -0.44285714 -0.42857143 -0.41428571 -0.4 -0.38571429 -0.37142857 -0.35714286 -0.34285714 -0.32857143 -0.31428571 -0.3 -0.28571429 -0.27142857 -0.25714286 -0.24285714 -0.22857143 -0.21428571 -0.2 -0.18571429 -0.17142857 -0.15714286 -0.14285714 -0.13777296 -0.13777296 -0.13777296 -0.13777296 -0.13777296 -0.13777296
  spline S143 degree 3 poles (6.1725, -26.3935) (6.1471, -26.3994) (6.1232, -26.4102) (6.0808, -26.4404) (6.0627, -26.4595) (6.038, -26.4988) (6.0299, -26.5175) (6.0195, -26.5568) (6.0173, -26.5771) (6.0183, -26.5974) knots 0 0 0 0 0.007813 0.007813 0.015626 0.015626 0.021719 0.021719 0.027811 0.027811 0.027811 0.027811
  arc A72 (6.1725, -26.3935) -> (6.941, -26.2019) centre (0, 0) ccw
  spline S144 degree 3 poles (7.1729, -26.3095) (7.1617, -26.286) (7.1461, -26.2648) (7.1076, -26.2298) (7.0851, -26.2162) (7.0415, -26.2003) (7.0215, -26.1963) (6.9809, -26.1945) (6.9606, -26.1967) (6.941, -26.2019) knots 0 0 0 0 0.007813 0.007813 0.015626 0.015626 0.021719 0.021719 0.027811 0.027811 0.027811 0.027811
  spline S145 degree 5 poles (7.1729, -26.3095) (7.1742, -26.3123) (7.1794, -26.3231) (7.1883, -26.3418) (7.2012, -26.3683) (7.2181, -26.4027) (7.2379, -26.4421) (7.258, -26.4813) (7.2785, -26.5205) (7.2992, -26.5595) (7.3203, -26.5984) (7.3417, -26.6372) (7.3634, -26.6759) (7.3854, -26.7145) (7.4076, -26.753) (7.4301, -26.7914) (7.4528, -26.8297) (7.4758, -26.8679) (7.4991, -26.906) (7.5226, -26.9441) (7.5463, -26.982) (7.5703, -27.0198) (7.5945, -27.0576) (7.619, -27.0952) (7.6436, -27.1328) (7.6685, -27.1702) (7.6937, -27.2076) (7.719, -27.2449) (7.7445, -27.2821) (7.7703, -27.3192) (7.7963, -27.3563) (7.8224, -27.3932) (7.8488, -27.4301) (7.8754, -27.4668) (7.9022, -27.5035) (7.9291, -27.5401) (7.9563, -27.5766) (7.9837, -27.6131) (8.0112, -27.6494) (8.0389, -27.6857) (8.0669, -27.7219) (8.095, -27.758) (8.1233, -27.794) (8.1517, -27.8299) (8.1804, -27.8658) (8.2092, -27.9015) (8.2382, -27.9372) (8.2674, -27.9728) (8.2968, -28.0083) (8.3263, -28.0438) (8.356, -28.0791) (8.3859, -28.1144) (8.4159, -28.1496) (8.4461, -28.1847) (8.4765, -28.2197) (8.507, -28.2547) (8.5377, -28.2895) (8.5686, -28.3243) (8.5996, -28.359) (8.6308, -28.3937) (8.6621, -28.4282) (8.6936, -28.4627) (8.7189, -28.4902) (8.738, -28.5108) (8.7507, -28.5245) (8.7571, -28.5313) knots 0.13777296 0.13777296 0.13777296 0.13777296 0.13777296 0.13777296 0.14285714 0.15714286 0.17142857 0.18571429 0.2 0.21428571 0.22857143 0.24285714 0.25714286 0.27142857 0.28571429 0.3 0.31428571 0.32857143 0.34285714 0.35714286 0.37142857 0.38571429 0.4 0.41428571 0.42857143 0.44285714 0.45714286 0.47142857 0.48571429 0.5 0.51428571 0.52857143 0.54285714 0.55714286 0.57142857 0.58571429 0.6 0.61428571 0.62857143 0.64285714 0.65714286 0.67142857 0.68571429 0.7 0.71428571 0.72857143 0.74285714 0.75714286 0.77142857 0.78571429 0.8 0.81428571 0.82857143 0.84285714 0.85714286 0.87142857 0.88571429 0.9 0.91428571 0.92857143 0.94285714 0.95714286 0.97142857 0.98571429 1 1 1 1 1 1
  arc A73 (8.7571, -28.5313) -> (9.6856, -28.2296) centre (0, 0) ccw
  spline S146 degree 5 poles (9.6856, -28.2296) (9.6868, -28.2203) (9.689, -28.2018) (9.6923, -28.1739) (9.6967, -28.1368) (9.7019, -28.0904) (9.7069, -28.044) (9.7118, -27.9977) (9.7165, -27.9514) (9.721, -27.9051) (9.7254, -27.8588) (9.7295, -27.8126) (9.7335, -27.7664) (9.7373, -27.7202) (9.7409, -27.6741) (9.7443, -27.628) (9.7476, -27.582) (9.7506, -27.5359) (9.7535, -27.4899) (9.7562, -27.444) (9.7587, -27.3981) (9.761, -27.3522) (9.7631, -27.3063) (9.765, -27.2605) (9.7667, -27.2148) (9.7683, -27.169) (9.7696, -27.1234) (9.7707, -27.0777) (9.7716, -27.0321) (9.7724, -26.9866) (9.7729, -26.9411) (9.7732, -26.8956) (9.7733, -26.8502) (9.7732, -26.8048) (9.7728, -26.7595) (9.7723, -26.7142) (9.7715, -26.669) (9.7706, -26.6238) (9.7694, -26.5787) (9.7679, -26.5336) (9.7663, -26.4886) (9.7644, -26.4437) (9.7623, -26.3988) (9.7599, -26.354) (9.7573, -26.3092) (9.7545, -26.2645) (9.7514, -26.2199) (9.7481, -26.1753) (9.7445, -26.1308) (9.7407, -26.0863) (9.7365, -26.042) (9.7322, -25.9977) (9.7275, -25.9535) (9.7226, -25.9094) (9.7174, -25.8653) (9.7119, -25.8213) (9.7061, -25.7775) (9.6999, -25.7337) (9.6934, -25.69) (9.6866, -25.6464) (9.6795, -25.6029) (9.673, -25.5652) (9.6678, -25.5361) (9.6641, -25.5157) (9.6619, -25.504) (9.6613, -25.5009) knots -1 -1 -1 -1 -1 -1 -0.98571429 -0.97142857 -0.95714286 -0.94285714 -0.92857143 -0.91428571 -0.9 -0.88571429 -0.87142857 -0.85714286 -0.84285714 -0.82857143 -0.81428571 -0.8 -0.78571429 -0.77142857 -0.75714286 -0.74285714 -0.72857143 -0.71428571 -0.7 -0.68571429 -0.67142857 -0.65714286 -0.64285714 -0.62857143 -0.61428571 -0.6 -0.58571429 -0.57142857 -0.55714286 -0.54285714 -0.52857143 -0.51428571 -0.5 -0.48571429 -0.47142857 -0.45714286 -0.44285714 -0.42857143 -0.41428571 -0.4 -0.38571429 -0.37142857 -0.35714286 -0.34285714 -0.32857143 -0.31428571 -0.3 -0.28571429 -0.27142857 -0.25714286 -0.24285714 -0.22857143 -0.21428571 -0.2 -0.18571429 -0.17142857 -0.15714286 -0.14285714 -0.13777296 -0.13777296 -0.13777296 -0.13777296 -0.13777296 -0.13777296
  spline S147 degree 3 poles (9.7857, -25.2775) (9.7614, -25.2869) (9.7392, -25.301) (9.7014, -25.3368) (9.6862, -25.3583) (9.6672, -25.4006) (9.6617, -25.4202) (9.6569, -25.4606) (9.6576, -25.481) (9.6613, -25.5009) knots 0 0 0 0 0.007813 0.007813 0.015626 0.015626 0.021719 0.021719 0.027811 0.027811 0.027811 0.027811
  arc A74 (9.7857, -25.2775) -> (10.52, -24.9809) centre (0, 0) ccw
  spline S148 degree 3 poles (10.7647, -25.0552) (10.7503, -25.0334) (10.7319, -25.0147) (10.6889, -24.9853) (10.6647, -24.975) (10.6194, -24.9653) (10.599, -24.9642) (10.5585, -24.968) (10.5387, -24.973) (10.52, -24.9809) knots 0 0 0 0 0.007813 0.007813 0.015626 0.015626 0.021719 0.021719 0.027811 0.027811 0.027811 0.027811
  spline S149 degree 5 poles (10.7647, -25.0552) (10.7664, -25.0578) (10.7729, -25.0677) (10.7844, -25.085) (10.8009, -25.1095) (10.8224, -25.1412) (10.8475, -25.1774) (10.8729, -25.2135) (10.8986, -25.2494) (10.9246, -25.2851) (10.9509, -25.3207) (10.9774, -25.3562) (11.0043, -25.3915) (11.0314, -25.4267) (11.0588, -25.4617) (11.0864, -25.4966) (11.1143, -25.5314) (11.1424, -25.566) (11.1707, -25.6005) (11.1992, -25.6349) (11.228, -25.6691) (11.2571, -25.7033) (11.2863, -25.7373) (11.3157, -25.7712) (11.3454, -25.8049) (11.3753, -25.8386) (11.4053, -25.8721) (11.4356, -25.9055) (11.4661, -25.9388) (11.4968, -25.9719) (11.5276, -26.005) (11.5587, -26.0379) (11.5899, -26.0708) (11.6214, -26.1035) (11.653, -26.1361) (11.6848, -26.1686) (11.7168, -26.201) (11.749, -26.2332) (11.7813, -26.2654) (11.8138, -26.2974) (11.8465, -26.3294) (11.8794, -26.3612) (11.9124, -26.3929) (11.9456, -26.4246) (11.979, -26.4561) (12.0125, -26.4875) (12.0462, -26.5188) (12.08, -26.55) (12.114, -26.5811) (12.1482, -26.612) (12.1825, -26.6429) (12.217, -26.6737) (12.2517, -26.7044) (12.2865, -26.7349) (12.3214, -26.7654) (12.3565, -26.7958) (12.3918, -26.826) (12.4272, -26.8562) (12.4627, -26.8862) (12.4984, -26.9162) (12.5343, -26.946) (12.5702, -26.9758) (12.5991, -26.9995) (12.6209, -27.0172) (12.6354, -27.029) (12.6427, -27.0349) knots 0.13777296 0.13777296 0.13777296 0.13777296 0.13777296 0.13777296 0.14285714 0.15714286 0.17142857 0.18571429 0.2 0.21428571 0.22857143 0.24285714 0.25714286 0.27142857 0.28571429 0.3 0.31428571 0.32857143 0.34285714 0.35714286 0.37142857 0.38571429 0.4 0.41428571 0.42857143 0.44285714 0.45714286 0.47142857 0.48571429 0.5 0.51428571 0.52857143 0.54285714 0.55714286 0.57142857 0.58571429 0.6 0.61428571 0.62857143 0.64285714 0.65714286 0.67142857 0.68571429 0.7 0.71428571 0.72857143 0.74285714 0.75714286 0.77142857 0.78571429 0.8 0.81428571 0.82857143 0.84285714 0.85714286 0.87142857 0.88571429 0.9 0.91428571 0.92857143 0.94285714 0.95714286 0.97142857 0.98571429 1 1 1 1 1 1
  arc A75 (12.6427, -27.0349) -> (13.5202, -26.6069) centre (0, 0) ccw
  spline S150 degree 5 poles (13.5202, -26.6069) (13.52, -26.5976) (13.5197, -26.5789) (13.5191, -26.5508) (13.5182, -26.5134) (13.5169, -26.4668) (13.5154, -26.4201) (13.5138, -26.3736) (13.512, -26.3271) (13.51, -26.2806) (13.5079, -26.2342) (13.5056, -26.1878) (13.5031, -26.1415) (13.5004, -26.0953) (13.4976, -26.0491) (13.4946, -26.003) (13.4914, -25.9569) (13.488, -25.9109) (13.4845, -25.865) (13.4807, -25.8191) (13.4768, -25.7733) (13.4727, -25.7275) (13.4684, -25.6818) (13.4639, -25.6362) (13.4593, -25.5907) (13.4544, -25.5452) (13.4494, -25.4997) (13.4441, -25.4544) (13.4387, -25.4091) (13.4331, -25.3639) (13.4272, -25.3187) (13.4212, -25.2737) (13.415, -25.2287) (13.4086, -25.1838) (13.4019, -25.1389) (13.3951, -25.0942) (13.3881, -25.0495) (13.3808, -25.0049) (13.3733, -24.9604) (13.3656, -24.916) (13.3577, -24.8716) (13.3496, -24.8274) (13.3413, -24.7832) (13.3327, -24.7392) (13.3239, -24.6952) (13.3149, -24.6513) (13.3056, -24.6075) (13.2961, -24.5639) (13.2864, -24.5203) (13.2764, -24.4768) (13.2661, -24.4335) (13.2556, -24.3902) (13.2449, -24.3471) (13.2339, -24.3041) (13.2226, -24.2612) (13.211, -24.2184) (13.1991, -24.1758) (13.187, -24.1333) (13.1745, -24.0909) (13.1617, -24.0487) (13.1486, -24.0067) (13.1369, -23.9701) (13.1277, -23.9421) (13.1211, -23.9224) (13.1174, -23.9111) (13.1164, -23.9082) knots -1 -1 -1 -1 -1 -1 -0.98571429 -0.97142857 -0.95714286 -0.94285714 -0.92857143 -0.91428571 -0.9 -0.88571429 -0.87142857 -0.85714286 -0.84285714 -0.82857143 -0.81428571 -0.8 -0.78571429 -0.77142857 -0.75714286 -0.74285714 -0.72857143 -0.71428571 -0.7 -0.68571429 -0.67142857 -0.65714286 -0.64285714 -0.62857143 -0.61428571 -0.6 -0.58571429 -0.57142857 -0.55714286 -0.54285714 -0.52857143 -0.51428571 -0.5 -0.48571429 -0.47142857 -0.45714286 -0.44285714 -0.42857143 -0.41428571 -0.4 -0.38571429 -0.37142857 -0.35714286 -0.34285714 -0.32857143 -0.31428571 -0.3 -0.28571429 -0.27142857 -0.25714286 -0.24285714 -0.22857143 -0.21428571 -0.2 -0.18571429 -0.17142857 -0.15714286 -0.14285714 -0.13777296 -0.13777296 -0.13777296 -0.13777296 -0.13777296 -0.13777296
  spline S151 degree 3 poles (13.2084, -23.6696) (13.1857, -23.6823) (13.1656, -23.6993) (13.1332, -23.7401) (13.1211, -23.7634) (13.1082, -23.8079) (13.1055, -23.8282) (13.1063, -23.8688) (13.1099, -23.8889) (13.1164, -23.9082) knots 0 0 0 0 0.007813 0.007813 0.015626 0.015626 0.021719 0.021719 0.027811 0.027811 0.027811 0.027811
  arc A76 (13.2084, -23.6696) -> (13.8943, -23.2736) centre (0, 0) ccw
  spline S152 degree 3 poles (14.1469, -23.3132) (14.1297, -23.2936) (14.1088, -23.2776) (14.0621, -23.2546) (14.0368, -23.2477) (13.9905, -23.2444) (13.9702, -23.2461) (13.9307, -23.2555) (13.9117, -23.2632) (13.8943, -23.2736) knots 0 0 0 0 0.007813 0.007813 0.015626 0.015626 0.021719 0.021719 0.027811 0.027811 0.027811 0.027811
  spline S153 degree 5 poles (14.1469, -23.3132) (14.149, -23.3155) (14.1569, -23.3245) (14.1706, -23.34) (14.1903, -23.3619) (14.2161, -23.3903) (14.246, -23.4227) (14.2761, -23.4549) (14.3066, -23.4869) (14.3373, -23.5187) (14.3683, -23.5503) (14.3995, -23.5817) (14.431, -23.6129) (14.4628, -23.6439) (14.4947, -23.6748) (14.527, -23.7055) (14.5594, -23.7361) (14.592, -23.7665) (14.6249, -23.7967) (14.6579, -23.8268) (14.6912, -23.8567) (14.7247, -23.8865) (14.7584, -23.9161) (14.7923, -23.9455) (14.8263, -23.9748) (14.8606, -24.004) (14.895, -24.033) (14.9297, -24.0618) (14.9645, -24.0906) (14.9995, -24.1191) (15.0346, -24.1476) (15.07, -24.1759) (15.1055, -24.204) (15.1412, -24.2321) (15.177, -24.2599) (15.2131, -24.2877) (15.2492, -24.3153) (15.2856, -24.3428) (15.3221, -24.3701) (15.3587, -24.3974) (15.3956, -24.4244) (15.4325, -24.4514) (15.4696, -24.4782) (15.5069, -24.5049) (15.5443, -24.5315) (15.5819, -24.5579) (15.6196, -24.5842) (15.6575, -24.6104) (15.6955, -24.6364) (15.7337, -24.6624) (15.772, -24.6882) (15.8104, -24.7138) (15.849, -24.7394) (15.8877, -24.7648) (15.9265, -24.7901) (15.9655, -24.8153) (16.0046, -24.8403) (16.0439, -24.8653) (16.0833, -24.8901) (16.1228, -24.9148) (16.1624, -24.9393) (16.2022, -24.9638) (16.2341, -24.9833) (16.2581, -24.9978) (16.2742, -25.0075) (16.2822, -25.0123) knots 0.13777296 0.13777296 0.13777296 0.13777296 0.13777296 0.13777296 0.14285714 0.15714286 0.17142857 0.18571429 0.2 0.21428571 0.22857143 0.24285714 0.25714286 0.27142857 0.28571429 0.3 0.31428571 0.32857143 0.34285714 0.35714286 0.37142857 0.38571429 0.4 0.41428571 0.42857143 0.44285714 0.45714286 0.47142857 0.48571429 0.5 0.51428571 0.52857143 0.54285714 0.55714286 0.57142857 0.58571429 0.6 0.61428571 0.62857143 0.64285714 0.65714286 0.67142857 0.68571429 0.7 0.71428571 0.72857143 0.74285714 0.75714286 0.77142857 0.78571429 0.8 0.81428571 0.82857143 0.84285714 0.85714286 0.87142857 0.88571429 0.9 0.91428571 0.92857143 0.94285714 0.95714286 0.97142857 0.98571429 1 1 1 1 1 1
  arc A77 (16.2822, -25.0123) -> (17.0916, -24.4663) centre (0, 0) ccw
  spline S154 degree 5 poles (17.0916, -24.4663) (17.0901, -24.4571) (17.0871, -24.4386) (17.0827, -24.4109) (17.0766, -24.374) (17.0688, -24.328) (17.0609, -24.282) (17.0528, -24.2361) (17.0445, -24.1903) (17.0361, -24.1446) (17.0275, -24.0989) (17.0188, -24.0534) (17.0099, -24.0079) (17.0008, -23.9624) (16.9916, -23.9171) (16.9822, -23.8719) (16.9726, -23.8267) (16.9629, -23.7816) (16.9529, -23.7366) (16.9429, -23.6917) (16.9326, -23.6469) (16.9222, -23.6021) (16.9115, -23.5575) (16.9008, -23.5129) (16.8898, -23.4684) (16.8787, -23.4241) (16.8673, -23.3798) (16.8558, -23.3356) (16.8442, -23.2915) (16.8323, -23.2475) (16.8202, -23.2036) (16.808, -23.1598) (16.7956, -23.1162) (16.783, -23.0726) (16.7702, -23.0291) (16.7572, -22.9857) (16.744, -22.9425) (16.7306, -22.8993) (16.717, -22.8563) (16.7032, -22.8134) (16.6892, -22.7706) (16.675, -22.7279) (16.6606, -22.6853) (16.646, -22.6429) (16.6312, -22.6005) (16.6161, -22.5583) (16.6008, -22.5163) (16.5854, -22.4744) (16.5696, -22.4326) (16.5537, -22.3909) (16.5375, -22.3494) (16.5211, -22.308) (16.5044, -22.2668) (16.4875, -22.2258) (16.4704, -22.1848) (16.453, -22.1441) (16.4353, -22.1035) (16.4173, -22.0631) (16.3991, -22.0229) (16.3805, -21.9829) (16.3617, -21.9431) (16.345, -21.9086) (16.332, -21.8821) (16.3228, -21.8635) (16.3175, -21.8529) (16.3161, -21.8501) knots -1 -1 -1 -1 -1 -1 -0.98571429 -0.97142857 -0.95714286 -0.94285714 -0.92857143 -0.91428571 -0.9 -0.88571429 -0.87142857 -0.85714286 -0.84285714 -0.82857143 -0.81428571 -0.8 -0.78571429 -0.77142857 -0.75714286 -0.74285714 -0.72857143 -0.71428571 -0.7 -0.68571429 -0.67142857 -0.65714286 -0.64285714 -0.62857143 -0.61428571 -0.6 -0.58571429 -0.57142857 -0.55714286 -0.54285714 -0.52857143 -0.51428571 -0.5 -0.48571429 -0.47142857 -0.45714286 -0.44285714 -0.42857143 -0.41428571 -0.4 -0.38571429 -0.37142857 -0.35714286 -0.34285714 -0.32857143 -0.31428571 -0.3 -0.28571429 -0.27142857 -0.25714286 -0.24285714 -0.22857143 -0.21428571 -0.2 -0.18571429 -0.17142857 -0.15714286 -0.14285714 -0.13777296 -0.13777296 -0.13777296 -0.13777296 -0.13777296 -0.13777296
  spline S155 degree 3 poles (16.3741, -21.601) (16.3533, -21.6168) (16.3358, -21.6364) (16.3094, -21.6813) (16.3006, -21.7061) (16.294, -21.7519) (16.2942, -21.7724) (16.3007, -21.8125) (16.307, -21.8319) (16.3161, -21.8501) knots 0 0 0 0 0.007813 0.007813 0.015626 0.015626 0.021719 0.021719 0.027811 0.027811 0.027811 0.027811
  arc A78 (16.3741, -21.601) -> (16.9981, -21.1134) centre (0, 0) ccw
  spline S156 degree 3 poles (17.2538, -21.1174) (17.234, -21.1005) (17.2111, -21.0875) (17.1617, -21.0712) (17.1356, -21.0679) (17.0894, -21.0711) (17.0694, -21.0756) (17.0316, -21.0904) (17.014, -21.1007) (16.9981, -21.1134) knots 0 0 0 0 0.007813 0.007813 0.015626 0.015626 0.021719 0.021719 0.027811 0.027811 0.027811 0.027811